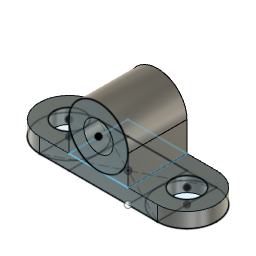
A4 (Autodesk Fusion 360 design; units mm, degrees)
Autodesk Fusion 360 part; units mm, degrees
note: some values were not read from the file. Set by a fixed rule: which sketch regions a step uses.
sketch "Sketch4" plane through (0, 0, 0) normal (0, 0, 1) x (1, 0, 0)
  line L0 (40, -20) -> (-40, -20)
  line L1 (-40, -20) -> (-40, 20)
  line L2 (-40, 20) -> (40, 20)
  line L3 (40, 20) -> (40, -20)
  line L4 (40, -20) -> (-40, 20) construction
  line L5 (-40, -20) -> (40, 20) construction
  circle A0 centre (40, 0) radius 20
  circle A1 centre (-40, 0) radius 20
  line L6 (-40, 20) -> (-20, 20)
  line L7 (-20, 20) -> (-20, -20)
  line L8 (-20, 20) -> (20, 20)
  line L9 (20, 20) -> (20, -20)
  dimension "d15" = 80
  dimension "d16" = 40
  dimension "d19" = 40
  dimension "d20" = 40
  dimension "d29" = 20
  dimension "d30" = 40
  constraint horizontal L0
  constraint perpendicular L0 L1
  constraint parallel L0 L2
  constraint parallel L1 L3
  constraint coincident L4 origin
  constraint coincident L5 origin
  constraint midpoint L3 A0.centre
  constraint midpoint L1 A1.centre
  constraint perpendicular L1 L6
  constraint coincident L0 L7.end
  constraint perpendicular L0 L7
  constraint perpendicular L7 L8
  constraint perpendicular L8 L9
  measures "d15" distance of L1.end L2.end
  measures "d16" distance of L0.end L1.end
  measures "d19" diameter of A0
  measures "d20" diameter of A1
  measures "d29" distance of L1.end L6.end
  measures "d30" distance of L6.end L8.end
extrude "Extrude3" add sketch "Sketch4" along normal blind 10
sketch "Sketch5" plane through (0, 0, 10) normal (0, 0, 1) x (-1, 0, 0)
  arc A0 (40, -20) -> (40, 20) centre (40, 0) ccw
  line L0 (40, 20) -> (-40, 20)
  arc A1 (-40, 20) -> (-40, -20) centre (-40, 0) ccw
  line L1 (-40, -20) -> (40, -20)
  circle A2 centre (40, 0) radius 10
  circle A3 centre (-40, 0) radius 10
  dimension "d23" = 20
  dimension "d24" = 20
  constraint concentric A0 A2
  constraint concentric A1 A3
  measures "d23" diameter of A2
  measures "d24" diameter of A3
extrude "Extrude4" cut sketch "Sketch5" against normal blind 10 contours A2
extrude "Extrude5" cut sketch "Sketch5" against normal blind 10 contours A3
sketch "Sketch7" plane through (0, 0, 10) normal (0, 0, 1) x (-1, 0, 0)
  line L0 (-20, 20) -> (20, 20)
  line L1 (20, 20) -> (20, -20)
  line L2 (20, -20) -> (-20, -20)
  line L3 (-20, -20) -> (-20, 20)
  dimension "d33" = 40
  dimension "d34" = 40
  constraint horizontal L0
  constraint vertical L1
  constraint horizontal L2
  constraint vertical L3
  measures "d33" distance of L0.start L0.end
  measures "d34" distance of L0.start L2.end
extrude "Extrude6" add sketch "Sketch7" along normal blind 20
sketch "Sketch8" plane through (0, -20, 0) normal (0, -1, 0) x (1, 0, 0)
  line L0 (-40, 0) -> (40, 0)
  line L1 (40, 0) -> (40, 10)
  line L2 (40, 10) -> (20, 10)
  line L3 (20, 10) -> (20, 30)
  line L4 (20, 30) -> (-20, 30)
  line L5 (-20, 30) -> (-20, 10)
  line L6 (-20, 10) -> (-40, 10)
  line L7 (-40, 10) -> (-40, 0)
  circle A0 centre (0, 30) radius 20
  dimension "d37" = 40
  constraint midpoint L4 A0.centre
  measures "d37" diameter of A0
extrude "Extrude7" add sketch "Sketch8" against normal blind 40 contours L4 A0 picked at (4.1566, 35.2122)
sketch "Sketch9" plane through (0, -20, 0) normal (0, -1, 0) x (1, 0, 0)
  circle A0 centre (0, 30) radius 10
  dimension "d40" = 20
  measures "d40" diameter of A0
extrude "Extrude8" cut sketch "Sketch9" against normal blind 40
